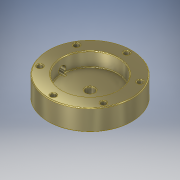
# Autodesk Inventor part: valvehousing
Saved by Autodesk Inventor 2017 (Build 210142000, 142)
## iProperties
Created: 2020-01-12
Part Number: valvehousing
Material: Gold
Document SubType Name: Modeling
Designer: Admin
Density: 19.3 g/cm^3
Appearance: Gold - Metal
Mass: 148.081 g
Surface Area: 44.3949 cm^2
Volume: 7.6726 cm^3
Author: Admin
Autodesk Inventor part; units mm, degrees
ref_plane "XZ Plane" through (0, 0, 0) normal (0, 1, 0) x (-1, 0, 0)
ref_plane "XY Plane" through (0, 0, 0) normal (0, 0, 1) x (1, 0, 0)
sketch "Sketch1" plane through (0, 0, 0) normal (0, 1, 0) x (-1, 0, 0)
  circle A0 centre (0, 0) radius 19.05
  dimension "d0" = 38.1
  constraints: 1 centre point, 1 coincident
  measures "d0" diameter of A0
extrude "Extrusion1" add sketch "Sketch1" along normal blind 9.525
sketch "Sketch2" plane through (0, 9.525, 0) normal (0, 1, 0) x (1, 0, 0)
  circle A0 centre (0, 0) radius 12.7
  dimension "d3" = 25.4
  constraints: 1 centre point, 1 coincident
  measures "d3" diameter of A0
extrude "Extrusion2" cut sketch "Sketch2" against normal blind 6.35
sketch "Sketch3" plane through (0, 3.175, 0) normal (0, 1, 0) x (1, 0, 0)
  point P0 (0, 0)
sketch "Sketch4" plane through (0, 0, 0) normal (0, -1, 0) x (1, 0, 0)
  circle A0 centre (0, 0) radius 1.9558
  circle A1 centre (0, 0) radius 6.35
  dimension "d6" = 3.9116
  dimension "d7" = 12.7
  constraints: 2 centre point, 2 coincident
  measures "d6" diameter of A0
  measures "d7" diameter of A1
extrude "Extrusion3" add sketch "Sketch4" along normal blind 3.175
extrude "Extrusion4" cut sketch "Sketch4" against normal blind 3.175 contours A0
sketch "Sketch5" plane through (0, 9.525, 0) normal (0, 1, 0) x (1, 0, 0)
  circle A0 centre (0, -16.6688) radius 1.1303
  circle A1 centre (0, 16.6688) radius 1.1303
  circle A2 centre (-14.4356, 8.3344) radius 1.1303
  circle A3 centre (-14.4356, -8.3344) radius 1.1303
  circle A4 centre (0, -16.6688) radius 1.1303
  circle A5 centre (14.4356, -8.3344) radius 1.1303
  circle A6 centre (14.4356, 8.3344) radius 1.1303
  point P0 (0, 0)
  dimension "d12" = 2.2606
  dimension "d13" = 2.2606
  dimension "d14" = 33.3375
  dimension "d15" = 16.6687
  dimension "d18" = 360
  constraints: 7 centre point, 13 other
  measures "d12" diameter of A0
  measures "d13" diameter of A1
  measures "d14" distance of A0.centre A1.centre
  measures "d15" distance of point (0, 0) A1.centre
extrude "Extrusion5" cut sketch "Sketch5" against normal through all
ref_plane "Work Plane1" through (-19.05, 0, 0) normal (1, 0, 0) x (0, 1, 0)
sketch "Sketch6" plane through (-19.05, 0, 0) normal (1, 0, 0) x (0, 1, 0)
  circle A0 centre (4.7625, 0) radius 1.6839
  line L0 (9.525, -19.05) -> (9.525, 19.05) projected
  line L1 (0, 19.05) -> (0, -19.05) projected
  line L2 (9.525, -19.05) -> (0, -19.05)
  point P0 (0, 0)
  point P1 (4.7625, -19.05)
  constraints: 2 end point, 1 centre point, 1 horizontal, 1 midpoint, 1 vertical alignment
extrude "Extrusion6" cut sketch "Sketch6" along normal blind 7.9375
thread "Thread1" size "6-32 UNC" class "2B" standard "ANSI Unified Screw Threads" length 5.08 offset 5.08
fillet "Fillet1" radius 0.3175 19 edges at (19.05, 0, 0) (19.05, 9.525, 0) (0.2809, 3.175, 12.6969) (0.2809, 3.175, -12.6969) (-12.7, 9.525, 0) (-18.9754, 4.7626, 1.6839) (-18.9754, 4.7623, -1.6839) (-15.5659, 9.525, 8.3344) (-1.1303, 9.525, 16.6688) (13.3053, 9.525, 8.3344) (13.3053, 9.525, -8.3344) (-1.1303, 9.525, -16.6688) (-15.5659, 9.525, -8.3344) (-6.35, -3.175, 0) (-1.9558, -3.175, 0) (-15.5659, 0, 8.3344) (-1.1303, 0, -16.6688) (-15.5659, 0, -8.3344) (-1.1303, 0, 16.6688)
fillet "Fillet2" radius 0.3175 3 edges at (13.3053, 0, 8.3344) (13.3053, 0, -8.3344) (-1.9558, 3.175, 0)
body "Solid1"
